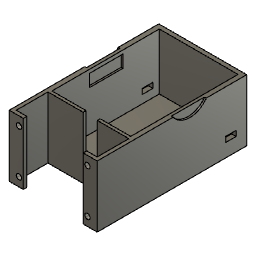
jbay_cover (Autodesk Fusion 360 design; units mm, degrees)
Autodesk Fusion 360 part; units mm, degrees
form "フォーム1" [no effect]
sketch "スケッチ5" plane through (0, 0, 0) normal (0, 1, 0) x (1, 0, 0)
  line L0 (0, 0) -> (50, 0)
  line L1 (50, 0) -> (50, -65)
  line L2 (50, -65) -> (0, -65)
  line L3 (0, -65) -> (0, 0)
  dimension "d9" = 50
  dimension "d10" = 65
  constraint horizontal L0
  constraint vertical L1
  constraint horizontal L2
  constraint vertical L3
  constraint coincident L0.start L3.end
  measures "d9" distance of L0.start L0.end
  measures "d10" distance of L0.start L2.end
extrude "押し出し4" add sketch "スケッチ5" along normal blind 35
sketch "スケッチ6" plane through (0, 35, 0) normal (0, 1, 0) x (-1, 0, 0)
  line L0 (0, 65) -> (-50, 65)
  line L1 (-50, 65) -> (-50, 0)
  line L2 (-50, 0) -> (0, 0)
  line L3 (0, 0) -> (0, 65)
  line L4 (-2.6641, 2.3571) -> (-47.4031, 2.3571)
  line L5 (-47.4031, 2.3571) -> (-47.4031, 63.3572)
  line L6 (-47.4031, 63.3572) -> (-2.6641, 63.3572)
  line L7 (-2.6641, 63.3572) -> (-2.6641, 2.3571)
  constraint horizontal L4
  constraint vertical L5
  constraint horizontal L6
  constraint vertical L7
extrude "押し出し5" cut sketch "スケッチ6" against normal blind 32 contours L4 L5 L6 L7
sketch "スケッチ7" plane through (0, 0, 0) normal (1, 0, 0) x (0, 0, -1)
  circle A0 centre (-32.5, 41.472) radius 11.4951
extrude "押し出し6" cut sketch "スケッチ7" along normal blind 1
sketch "スケッチ8" plane through (50, 0, 0) normal (1, 0, 0) x (0, 0, -1)
  line L0 (-65, 0) -> (0, 0)
  line L1 (0, 0) -> (0, 35)
  line L2 (0, 35) -> (-65, 35)
  line L3 (-65, 35) -> (-65, 0)
  circle A0 centre (-32.388, 41.5499) radius 11.5083
extrude "押し出し7" cut sketch "スケッチ8" against normal blind 1 contours L2 A0 picked at (-34.7651, 34.1724)
sketch "スケッチ9" plane through (2.6641, 0, 0) normal (1, 0, 0) x (0, 0, -1)
  line L0 (-2.3571, 35) -> (-63.3572, 35)
  line L1 (-63.3572, 35) -> (-63.3572, 3)
  line L2 (-63.3572, 3) -> (-2.3571, 3)
  line L3 (-2.3571, 3) -> (-2.3571, 35)
  line L4 (-42, 33) -> (-23, 33)
  line L5 (-23, 33) -> (-23, 26)
  line L6 (-23, 26) -> (-42, 26)
  line L7 (-42, 26) -> (-42, 33)
  dimension "d21" = 19
  dimension "d22" = 7
  constraint horizontal L4
  constraint vertical L5
  constraint horizontal L6
  constraint vertical L7
  measures "d21" distance of L4.start L4.end
  measures "d22" distance of L4.end L5.end
extrude "押し出し8" cut sketch "スケッチ9" against normal blind 1 contours L4 L5 L6 L7
sketch "スケッチ10" plane through (47.4031, 0, 0) normal (-1, 0, 0) x (0, 0, 1)
  line L0 (63.3572, 35) -> (2.3571, 35)
  line L1 (2.3571, 35) -> (2.3571, 3)
  line L2 (2.3571, 3) -> (63.3572, 3)
  line L3 (63.3572, 3) -> (63.3572, 35)
  line L4 (23, 33) -> (42, 33)
  line L5 (42, 33) -> (42, 26)
  line L6 (42, 26) -> (23, 26)
  line L7 (23, 26) -> (23, 33)
  constraint horizontal L4
  constraint vertical L5
  constraint horizontal L6
  constraint vertical L7
extrude "押し出し9" cut sketch "スケッチ10" against normal blind 1 contours L4 L5 L6 L7
sketch "スケッチ11" plane through (0, 35, 0) normal (0, 1, 0) x (-1, 0, 0)
sketch "スケッチ12" plane through (0, 0, 65) normal (0, 0, 1) x (1, 0, 0)
  line L0 (0, 0) -> (50, 0)
  line L1 (50, 0) -> (50, 35)
  line L2 (50, 35) -> (0, 35)
  line L3 (0, 35) -> (0, 0)
  line L4 (22, 35) -> (30, 35)
  line L5 (30, 35) -> (30, 12)
  line L6 (30, 12) -> (22, 12)
  line L7 (22, 12) -> (22, 35)
  line L8 (22.5, 11) -> (29.5, 11)
  line L9 (29.5, 11) -> (29.5, 12)
  line L10 (29.5, 12) -> (22.5, 12)
  line L11 (22.5, 12) -> (22.5, 11)
  dimension "d25" = 23
  dimension "d26" = 7
  dimension "d27" = 1
  constraint horizontal L4
  constraint vertical L5
  constraint horizontal L6
  constraint vertical L7
  constraint horizontal L8
  constraint vertical L9
  constraint horizontal L10
  constraint vertical L11
  measures "d25" distance of L4.end L5.end
  measures "d26" distance of L8.start L8.end
  measures "d27" distance of L8.start L10.end
extrude "押し出し10" cut sketch "スケッチ12" against normal blind 4 contours L2 L4 L5 L6 L7 L10 | L6 L8 L9 L10 L11
sketch "スケッチ13" plane through (0, 35, 0) normal (0, 1, 0) x (-1, 0, 0)
sketch "スケッチ14" plane through (0, 0, 0) normal (1, 0, 0) x (0, 0, -1)
  line L0 (-6, 10.6) -> (-12, 10.6)
  line L1 (-12, 10.6) -> (-12, 7.6)
  line L2 (-12, 7.6) -> (-6, 7.6)
  line L3 (-6, 7.6) -> (-6, 10.6)
  dimension "d30" = 6
  dimension "d33" = 3
  constraint horizontal L0
  constraint vertical L1
  constraint horizontal L2
  constraint vertical L3
  measures "d30" distance of L0.start L0.end
  measures "d33" distance of L0.end L1.end
extrude "押し出し11" cut sketch "スケッチ14" along normal blind 50
sketch "スケッチ15" plane through (0, 0, 65) normal (0, 0, 1) x (1, 0, 0)
  line L0 (0, 35) -> (2, 35)
  line L1 (2, 35) -> (2, 0)
  line L2 (2, 0) -> (0, 0)
  line L3 (0, 0) -> (0, 35)
  line L4 (48, 35) -> (50, 35)
  line L5 (50, 35) -> (50, 0)
  line L6 (50, 0) -> (48, 0)
  line L7 (48, 0) -> (48, 35)
  constraint horizontal L0
  constraint vertical L1
  constraint horizontal L2
  constraint vertical L3
  constraint horizontal L4
  constraint vertical L5
  constraint horizontal L6
  constraint vertical L7
extrude "押し出し12" add sketch "スケッチ15" along normal blind 20
sketch "スケッチ16" plane through (2, 0, 0) normal (1, 0, 0) x (0, 0, -1)
  line L0 (-65, 0) -> (-65, 35)
  line L1 (-65, 35) -> (-85, 35)
  line L2 (-85, 35) -> (-85, 0)
  line L3 (-85, 0) -> (-65, 0)
  line L4 (-85, 35) -> (-83, 35)
  line L5 (-83, 35) -> (-83, 0)
  line L6 (-83, 0) -> (-85, 0)
  line L7 (-85, 0) -> (-85, 35)
  constraint horizontal L4
  constraint vertical L5
  constraint horizontal L6
  constraint vertical L7
  constraint coincident L1.end L2.start
extrude "押し出し13" add sketch "スケッチ16" along normal blind 6 contours L1 L2 L3 L4 L5 L6 L7
sketch "スケッチ17" plane through (48, 0, 0) normal (-1, 0, 0) x (0, 0, 1)
  line L0 (65, 35) -> (65, 0)
  line L1 (65, 0) -> (85, 0)
  line L2 (85, 0) -> (85, 35)
  line L3 (85, 35) -> (65, 35)
  line L4 (83, 35) -> (85, 35)
  line L5 (85, 35) -> (85, 0)
  line L6 (85, 0) -> (83, 0)
  line L7 (83, 0) -> (83, 35)
  constraint horizontal L4
  constraint vertical L5
  constraint horizontal L6
  constraint vertical L7
  constraint coincident L1.end L2.start
  constraint coincident L3 L4.start
extrude "押し出し14" add sketch "スケッチ17" along normal blind 6 contours L1 L2 L3 L4 L5 L6 L7
hole "穴1" at (4.2693, 29.1043, 85) direction (0, 0, -1) diameter 2 depth 2 tip angle 118
hole "穴2" at (4.0834, 5.5355, 85) direction (0, 0, -1) diameter 2 depth 2 tip angle 118
hole "穴3" at (46.3415, 28.2261, 85) direction (0, 0, -1) diameter 2 depth 2 tip angle 118
hole "穴4" at (46.3546, 5.5927, 85) direction (0, 0, -1) diameter 2 depth 2 tip angle 118
move_face "面を移動1" to x (1, 0, 0) y (0, 1, 0) z (0, 0, 1) at (-1, 0, 0) 1 faces at (46.73, 29.1476, 84.3333)
move_face "面を移動2" to x (1, 0, 0) y (0, 1, 0) z (0, 0, 1) at (-1, 0, 0) 1 faces at (45.9662, 4.6712, 84.3333)
move_face "面を移動3" to x (1, 0, 0) y (0, 1, 0) z (0, 0, 1) at (1, 0, 0) 1 faces at (4.3689, 28.1093, 83.6667)
move_face "面を移動4" to x (1, 0, 0) y (0, 1, 0) z (0, 0, 1) at (1, 0, 0) 1 faces at (4.1333, 4.5367, 84.3333)
sketch "スケッチ18" plane through (0, 0, 85) normal (0, 0, 1) x (1, 0, 0)
  circle A0 centre (5.0834, 5.5355) radius 1
  circle A1 centre (5.2693, 29.1043) radius 1
  line L0 (0, 0) -> (8, 0)
  line L1 (8, 0) -> (8, 35)
  line L2 (8, 35) -> (0, 35)
  line L3 (0, 35) -> (0, 0)
  circle A2 centre (5.2693, 29.1043) radius 1.5
  dimension "d52" = 3
  constraint concentric A1 A2
  measures "d52" diameter of A2
extrude "押し出し15" cut sketch "スケッチ18" against normal blind 5 contours A1 | A2
sketch "スケッチ19" plane through (0, 0, 65) normal (0, 0, 1) x (1, 0, 0)
  line L0 (48, 0) -> (48, 35)
  line L1 (48, 35) -> (30, 35)
  line L2 (30, 35) -> (30, 12)
  line L3 (30, 12) -> (29.5, 12)
  line L4 (29.5, 12) -> (29.5, 11)
  line L5 (29.5, 11) -> (22.5, 11)
  line L6 (22.5, 11) -> (22.5, 12)
  line L7 (22.5, 12) -> (22, 12)
  line L8 (22, 12) -> (22, 35)
  line L9 (22, 35) -> (2, 35)
  line L10 (2, 35) -> (2, 0)
  line L11 (2, 0) -> (48, 0)
sketch "スケッチ20" plane through (0, 0, 85) normal (0, 0, 1) x (1, 0, 0)
  circle A0 centre (5.2693, 29.1043) radius 1.5
  circle A1 centre (5.0834, 5.5355) radius 1
  line L0 (0, 0) -> (8, 0)
  line L1 (8, 0) -> (8, 35)
  line L2 (8, 35) -> (0, 35)
  line L3 (0, 35) -> (0, 0)
hole "穴5" at (5.0834, 5.5355, 85) direction (0, 0, -1) diameter 3 depth 2 tip angle 118
hole "穴6" at (45.3415, 28.2261, 85) direction (0, 0, -1) diameter 3 depth 3 tip angle 118
hole "穴7" at (45.3546, 5.5927, 85) direction (0, 0, -1) diameter 3 depth 3 tip angle 118
sketch "スケッチ21" plane through (0, 0, 65) normal (0, 0, 1) x (1, 0, 0)
  line L0 (-1, 30) -> (51, 30)
  line L1 (-1, 5) -> (51, 5)
  line L2 (5.5501, 35.9938) -> (5.5501, -1)
  line L3 (44.4789, 35.9483) -> (44.4789, -1)
  circle A0 centre (5.5501, 30) radius 1.5
  circle A1 centre (44.4789, 30) radius 1.5
  circle A2 centre (5.5501, 5) radius 1.5
  circle A3 centre (44.4789, 5) radius 1.5
  dimension "d64" = 3
  dimension "d65" = 3
  dimension "d66" = 3
  dimension "d67" = 3
  constraint horizontal L0
  constraint horizontal L1
  constraint perpendicular L1 L2
  constraint perpendicular L1 L3
  constraint coincident L0 A0.centre
  constraint coincident L2 A0.centre
  constraint coincident L0 A1.centre
  constraint coincident L3 A1.centre
  constraint coincident L1 A2.centre
  constraint coincident L2 A2.centre
  constraint coincident L1 A3.centre
  constraint coincident L3 A3.centre
  measures "d64" diameter of A0
  measures "d65" diameter of A1
  measures "d66" diameter of A2
  measures "d67" diameter of A3
sketch "スケッチ22" plane through (0, 0, 85) normal (0, 0, 1) x (1, 0, 0)
  circle A0 centre (5.0834, 5.5355) radius 1.5
  circle A1 centre (5.2693, 29.1043) radius 1.5
  line L0 (0, 0) -> (8, 0)
  line L1 (8, 0) -> (8, 35)
  line L2 (8, 35) -> (0, 35)
  line L3 (0, 35) -> (0, 0)
extrude "押し出し16" add sketch "スケッチ22" against normal blind 2 contours A1
delete_face "面を削除2" 1 faces at (5.2328, 4.0429, 83.6667)
delete_face "面を削除3" 1 faces at (45.8546, 26.8166, 84.3333)
delete_face "面を削除4" 1 faces at (45.8676, 4.1831, 84.3333)
extrude "押し出し17" cut sketch "スケッチ21" along normal blind 27 contours L1 L3 A3 | L1 L3 A3 | L1 L3 A3 | L1 L3 A3
extrude "押し出し18" cut sketch "スケッチ21" along normal blind 26 contours L0 L2 A0 | L0 L2 A0 | L0 L2 A0 | L0 L2 A0 | L1 L2 A2 | L1 L2 A2 | L0 L3 A1 | L0 L3 A1 | L1 L2 A2 | L1 L2 A2 | L0 L3 A1 | L0 L3 A1
